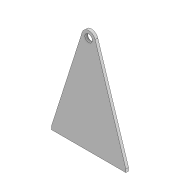
# Autodesk Inventor part: mount
Saved by Autodesk Inventor 2020 (Build 240168000, 168)
## iProperties
Created: 2021-06-21
Part Number: mount
Material: Generic
Document SubType Name: Modeling
Designer: Aidan Lee
Density: 1 g/cm^3
Appearance: Default
Author: Aidan Lee
Autodesk Inventor part; units mm, degrees
ref_plane "YZ Plane" through (0, 0, 0) normal (1, 0, 0) x (0, 1, 0)
ref_plane "XZ Plane" through (0, 0, 0) normal (0, 1, 0) x (-1, 0, 0)
ref_plane "XY Plane" through (0, 0, 0) normal (0, 0, 1) x (1, 0, 0)
sketch "Sketch1" plane through (0, 0, 0) normal (0, 0, 1) x (1, 0, 0)
  line L0 (0, 0) -> (220, 0)
  line L1 (220, 0) -> (220, 9)
  line L2 (220, 9) -> (0, 9)
  line L3 (0, 9) -> (0, 0)
  line L4 (0, 9) -> (90.94, 295.0593)
  line L5 (129.06, 295.0593) -> (220, 9)
  circle A0 centre (110, 289) radius 11
  line L6 (96.1101, 281.616) -> (103.5522, 305.0259) construction
  arc A1 (129.06, 295.0593) -> (90.94, 295.0593) centre (110, 289) ccw
  point P0 (110, 0)
  dimension "d0" = 9
  dimension "d1" = 220
  dimension "d2" = 22
  dimension "d3" = 280
  dimension "d4" = 9
  constraints: 14 end point, 3 parallel, 3 tangent, 2 centre point, 2 point on circle, 1 coincident, 1 horizontal, 1 midpoint, 1 perpendicular, 1 vertical alignment
  measures "d0" distance of L2.end L0.start
  measures "d1" distance of L0.start L0.end
  measures "d2" diameter of A0
  measures "d3" distance from line of L2 A0.centre
  measures "d4" distance between parallel lines of L4 L6
extrude "Extrusion1" add sketch "Sketch1" along normal blind 8
body "Solid1"
